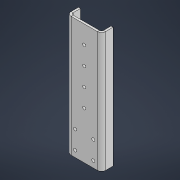
# Autodesk Inventor part: Bed Mount
Saved by Autodesk Inventor 2022 (Build 260153000, 153)
## iProperties
Created: 2021-10-05
Part Number: Bed Mount
Material: Generic
Document SubType Name: Sheet Metal
Designer: Administrator
Density: 1 g/cm^3
Appearance: Default
Sheet Metal Rule: .090 Steel
Sheet Metal Width: 55.454 mm
Sheet Metal Length: 132.000 mm
Sheet Metal Area: 7319.878 mm^2
Flat Pattern Width: 5.54536 cm
Flat Pattern Length: 13.2 cm
Flat Pattern Area: 73.1988 cm^2
Title: Bed Mount v4
Author: Administrator
Autodesk Inventor part; units mm, degrees
ref_plane "YZ Plane" through (0, 0, 0) normal (1, 0, 0) x (0, 1, 0)
ref_plane "XZ Plane" through (0, 0, 0) normal (0, 1, 0) x (-1, 0, 0)
ref_plane "XY Plane" through (0, 0, 0) normal (0, 0, 1) x (1, 0, 0)
sketch "Sketch1" plane through (0, 0, 0) normal (0, 0, 1) x (1, 0, 0)
  line L0 (0, 0) -> (-38, 0)
  line L1 (-38, 0) -> (-38, -132)
  line L2 (-38, -132) -> (0, -132)
  line L3 (0, -132) -> (0, 0)
  line L4 (-29, -105) -> (-9, -105) construction
  line L5 (-9, -105) -> (-9, -125) construction
  line L6 (-9, -125) -> (-29, -125) construction
  line L7 (-29, -125) -> (-29, -105) construction
  line L8 (-19, -105) -> (-19, -80) construction
  line L9 (-19, -80) -> (-19, -60) construction
  line L10 (-19, -60) -> (-19, -40) construction
  line L11 (-19, -40) -> (-19, -20) construction
  line L12 (-19, -20) -> (-19, 0) construction
  dimension "d0" = 20
  dimension "d1" = 20
  dimension "d2" = 25
  dimension "d3" = 20
  dimension "d4" = 7
  dimension "d5" = 9
  constraints: 26 end point, 6 collinear, 4 coincident, 4 parallel, 2 horizontal, 2 midpoint, 2 perpendicular, 2 vertical
  measures "d0" distance of L5.end L6.end
  measures "d1" distance of L6.end L4.start
  measures "d2" distance of L8.start L8.end
  measures "d3" distance of L8.end L9.end
  measures "d4" distance between parallel lines of L2 L6
  measures "d5" distance between parallel lines of L7 L1
extrude "Plate1" add sketch "Sketch1" along normal blind 2.286
hole "Hole1" at (-19, -80, 0) at (-19, -60, 0) at (-19, -40, 0) at (-19, -20, 0) at (-9, -125, 0) at (-9, -105, 0) at (-29, -105, 0) at (-29, -125, 0) direction (0, 0, 1) diameter 3.4 end through all clearance for "Socket Head Cap Screw" size "M3" standard "Ansi Metric M Profile"
sketch "Sketch2" plane through (-35.714, 0, 2.286) normal (-1, 0, 0) x (0, -1, 0)
  line L0 (132, 0) -> (0, 0)
  line L1 (0, 0) -> (0, -12.7)
  line L2 (0, -12.7) -> (132, -12.7)
  line L3 (132, -12.7) -> (132, 0)
  constraints: 6 end point, 1 horizontal, 1 perpendicular, 1 vertical
edge flange "Flange1" height 12.7 angle 90 thickness 2.286 bend radius 2.286 thickness toward (-1, 0, 0) relief straight relief width 2.286 relief depth 1.143 corner gap 2.286 corner form 0 edges at (-38, -66, 0) (0, -66, 0) wall of the first edge with corners at (-35.714, -132, 2.286) (-35.714, 0, 2.286) (-35.714, 0, -10.414) (-35.714, -132, -10.414)
bend "Bend1"
corner "Corner1"
equation "\"d12\" = Thickness"
equation "\"d6\" = Thickness"
equation "\"d14\" = BendReliefWidth"
equation "\"d15\" = BendReliefDepth"
equation "\"d16\" = MinimumRemnant"
equation "\"d17\" = TransitionRadius"
equation "\"d20\" = BendRadius"
equation "\"d21\" = CornerReliefSize"
equation "\"d22\" = GapSize"
equation "\"d23\" = JacobiRadiusSize"
equation "\"BendRadius\" = Thickness"
equation "\"BendReliefWidth\" = Thickness"
equation "\"BendReliefDepth\" = 0.5 * Thickness"
equation "\"CornerReliefSize\" = 4 * Thickness"
equation "\"MinimumRemnant\" = 2 * Thickness"
equation "\"TransitionRadius\" = BendRadius"
equation "\"JacobiRadiusSize\" = BendRadius"
equation "\"GapSize\" = Thickness"
equation "\"Thickness\" = 2.286"
body "Solid1"
body "Solid2"
